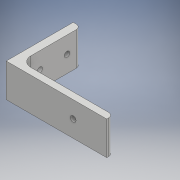
# Autodesk Inventor part: L_ShapedBracket_100x200x10_ozce
Saved by Autodesk Inventor 2017 (Build 210142000, 142)
## iProperties
Created: 2016-12-25
Part Number: L_ShapedBracket_100x200x10_ozce
Material: Generic
Document SubType Name: Modeling
Designer: umr
Density: 1 g/cm^3
Appearance: Default
Author: umr
Autodesk Inventor part; units mm, degrees
ref_plane "YZ Plane" through (0, 0, 0) normal (1, 0, 0) x (0, 1, 0)
ref_plane "XZ Plane" through (0, 0, 0) normal (0, 1, 0) x (-1, 0, 0)
ref_plane "XY Plane" through (0, 0, 0) normal (0, 0, 1) x (1, 0, 0)
sketch "Sketch1" plane through (0, 0, 0) normal (0, 1, 0) x (-1, 0, 0)
  line L0 (0, 0) -> (150, 0)
  line L1 (150, 0) -> (150, -50)
  line L2 (150, -50) -> (0, -50)
  line L3 (0, -50) -> (0, 0)
  dimension "d0" = 150
  dimension "d1" = 50
  constraints: 8 end point, 2 parallel, 1 horizontal, 1 perpendicular
  measures "d0" distance of L1.end L2.end
  measures "d1" distance of L0.end L1.end
extrude "Extrusion1" add sketch "Sketch1" along normal blind 10
sketch "Sketch2" plane through (0, 10, 0) normal (0, 1, 0) x (1, 0, 0)
  line L0 (-150, 50) -> (-150, 0) projected
  line L1 (-150, 0) -> (-138.3436, 0)
  line L2 (-138.3436, 0) -> (-138.3436, 50)
  line L3 (-138.3436, 50) -> (-150, 50)
  line L4 (-150, 50) -> (-150, 0)
  point P0 (0, 0)
  constraints: 8 end point, 2 parallel, 1 horizontal, 1 perpendicular
extrude "Extrusion2" add sketch "Sketch2" along normal blind 90
fillet "Fillet1" radius 15 1 edges at (-138.3436, 10, -25)
fillet "Fillet2" radius 7.5 2 edges at (-138.3436, 100, -25) (0, 10, -25)
sketch "Sketch3" plane through (-138.3436, 25, 0) normal (1, 0, 0) x (0, 0, -1)
  line L0 (0, 0) -> (0, 67.5) projected
  line L1 (50, 0) -> (50, 67.5) projected
  line L2 (0, 67.5) -> (50, 67.5) projected
  line L3 (0, 0) -> (0, 67.5) projected
  line L4 (50, 0) -> (0, 0) projected
  line L5 (50, 0) -> (50, 67.5) projected
  circle A0 centre (25, 54) radius 4
  circle A1 centre (25, 13.5) radius 4
  point P0 (0, -25)
  dimension "d8" = 8
  dimension "d9" = 8
  dimension "d10" = 67.5
  dimension "d11" = 50
  dimension "d12" = 25
  dimension "d13" = 13.5
  dimension "d14" = 13.5
  dimension "d17" = 40.5
  constraints: 2 centre point
  measures "d8" diameter of A0
  measures "d9" diameter of A1
  measures "d10" distance of L0.start L0.end
  measures "d11" distance of L2.start L2.end
  measures "d12" distance from line of L0 A0.centre
  measures "d13" distance from line of L2 A0.centre
  measures "d14" distance from line of L4 A1.centre
  measures "d17" distance of A1.centre A0.centre
extrude "Extrusion3" cut sketch "Sketch3" against normal up to next contours A0 | A1
sketch "Sketch4" plane through (0, 0, 0) normal (0, -1, 0) x (1, 0, 0)
  line L0 (-150, 0) -> (-150, -50) projected
  circle A0 centre (-50, -25) radius 4.25
  line L1 (0, 0) -> (-150, 0) projected
  dimension "d18" = 8.5
  dimension "d19" = 100
  dimension "d20" = 50
  dimension "d21" = 25
  constraints: 1 centre point
  measures "d18" diameter of A0
  measures "d19" distance from line of L0 A0.centre
  measures "d20" distance of L0.start L0.end
  measures "d21" distance from line of L1 A0.centre
extrude "Extrusion4" cut sketch "Sketch4" against normal blind 10
equation "\"d12\" = 0.5 * d11"
equation "\"d13\" = 0.2 * d10"
equation "\"d14\" = d13"
equation "\"d21\" = 0.5 * d20"
body "Solid1"
